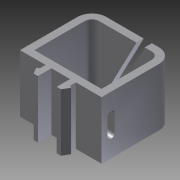
# Autodesk Inventor part: Cable V3
Saved by Autodesk Inventor 2012 (Build 160160000, 160)
## iProperties
Created: 2013-02-21
Part Number: Cable V3
Material: Default
Document SubType Name: Modeling
Designer: mce
Density: 1 g/cm^3
Author: mce
Autodesk Inventor part; units mm, degrees
ref_plane "YZ Plane" through (0, 0, 0) normal (1, 0, 0) x (0, 1, 0)
ref_plane "XZ Plane" through (0, 0, 0) normal (0, 1, 0) x (-1, 0, 0)
ref_plane "XY Plane" through (0, 0, 0) normal (0, 0, 1) x (1, 0, 0)
sketch "Sketch1" plane through (0, 0, 0) normal (0, 0, 1) x (1, 0, 0)
  line L0 (-0.3861, 13.3644) -> (-0.3861, 12.1644)
  line L1 (0.8139, 10.5644) -> (0.8139, 13.3644)
  line L2 (2.7639, 27.7657) -> (2.7639, 5.268) construction
  line L3 (-5.7361, 13.3644) -> (-5.7361, 25.3644)
  line L4 (-2.7361, 28.3644) -> (2.7639, 28.3644)
  line L5 (2.7639, 26.8644) -> (-2.7361, 26.8644)
  line L6 (-4.2361, 25.3644) -> (-4.2361, 14.8644)
  line L7 (-4.2361, 14.8644) -> (2.7639, 14.8644)
  line L8 (-0.3861, 12.1644) -> (-0.8539, 11.8943)
  line L9 (-5.7361, 13.3644) -> (-0.3861, 13.3644)
  arc A0 (-2.7361, 28.3644) -> (-5.7361, 25.3644) centre (-2.7361, 25.3644) ccw
  arc A1 (-2.7361, 26.8644) -> (-4.2361, 25.3644) centre (-2.7361, 25.3644) ccw
  line L10 (-0.8539, 11.8943) -> (-0.0861, 10.5644)
  line L11 (-0.0861, 10.5644) -> (0.8139, 10.5644)
  line L12 (5.6139, 10.5644) -> (4.7139, 10.5644)
  line L13 (11.2639, 13.3644) -> (11.2639, 25.3644)
  arc A2 (11.2639, 25.3644) -> (8.2639, 28.3644) centre (8.2639, 25.3644) ccw
  line L14 (8.2639, 28.3644) -> (2.7639, 28.3644)
  line L15 (2.7639, 26.8644) -> (8.2639, 26.8644)
  arc A3 (9.7639, 25.3644) -> (8.2639, 26.8644) centre (8.2639, 25.3644) ccw
  line L16 (9.7639, 25.3644) -> (9.7639, 14.8644)
  line L17 (9.7639, 14.8644) -> (2.7639, 14.8644)
  line L18 (11.2639, 13.3644) -> (5.9139, 13.3644)
  line L19 (5.9139, 13.3644) -> (5.9139, 12.1644)
  line L20 (5.9139, 13.3644) -> (6.9559, 13.3644)
  line L21 (4.7139, 10.5644) -> (4.7139, 13.3644)
  line L22 (6.3817, 11.8943) -> (5.6139, 10.5644)
  line L23 (5.9139, 12.1644) -> (6.3817, 11.8943)
  line L24 (0.8139, 13.3644) -> (4.7139, 13.3644)
  line L25 (5.9139, 13.3644) -> (6.9559, 13.3644)
  point P0 (0, 0)
  dimension "d1" = 1.2
  dimension "d2" = 1.95
  dimension "d3" = 120
  dimension "d5" = 8.5
  dimension "d6" = 1.5
  dimension "d8" = 1.5
  dimension "d9" = 12
  dimension "d10" = 3
  dimension "d11" = 1.5
  dimension "d12" = 0.9
  dimension "d13" = 120
  dimension "d15" = 1.2
  dimension "d16" = 2.8
  dimension "d17" = 1.5
  constraints: 52 end point, 14 symmetric about line, 8 point on circle, 4 centre point, 4 tangent, 3 horizontal, 3 point on line, 2 parallel, 2 vertical, 1 collinear, 1 perpendicular, 2 other
  measures "d1" distance between parallel lines of L0 L1
  measures "d2" distance between parallel lines of L2 L1
  measures "d3" angle of L0 L8
  measures "d5" distance between parallel lines of L2 L3
  measures "d6" distance between parallel lines of L3 L6
  measures "d8" distance between parallel lines of L4 L5
  measures "d9" distance between parallel lines of L5 L7
  measures "d10" radius of A0
  measures "d11" radius of A1
  measures "d12" distance of L11.start L1.start
  measures "d13" angle of L10 L11
  measures "d15" distance from line of L9 L8.start
  measures "d16" distance between parallel lines of L24 L11
  measures "d17" distance between parallel lines of L7 L9
extrude "Extrusion1" add sketch "Sketch1" along normal blind 12
sketch "Sketch2" plane through (-2.7361, 28.3644, 0) normal (0, 1, 0) x (1, 0, 0)
  line L0 (0, -12) -> (11, -12) projected
  line L1 (11, 0) -> (0, 0) projected
  line L2 (0, 0) -> (0, -12) projected
  line L3 (1.5, 0) -> (3.1945, 0)
  line L4 (3.1945, 0) -> (9.5, -12)
  line L5 (7.8055, -12) -> (1.5, 0)
  point P0 (2.7361, 0)
  dimension "d20" = 1.5
  dimension "d21" = 1.5
  dimension "d22" = 1.5
  constraints: 6 end point, 4 point on line, 1 parallel
  measures "d20" distance from line of L2 L3.start
  measures "d21" distance of L4.end L0.end
  measures "d22" distance between parallel lines of L5 L4
extrude "Extrusion2" cut sketch "Sketch2" against normal up to next contours L5 L1 L4 L0
sketch "Sketch3" plane through (11.2639, 13.3644, 0) normal (1, 0, 0) x (0, 0, -1)
  line L0 (-12, 12) -> (-12, 0) projected
  line L1 (0, 0) -> (-12, 0) projected
  arc A0 (-7.75, 2.75) -> (-7.75, 1.25) centre (-7.75, 2) ccw
  arc A1 (-4.25, 1.25) -> (-4.25, 2.75) centre (-4.25, 2) ccw
  line L2 (-7.75, 2.75) -> (-4.25, 2.75)
  line L3 (-4.25, 1.25) -> (-7.75, 1.25)
  point P0 (0, -13.3644)
  dimension "d30" = 1.5
  dimension "d31" = 3.5
  dimension "d32" = 4.25
  dimension "d33" = 2
  constraints: 4 end point, 4 point on circle, 4 vertical alignment, 2 centre point, 1 equal radius, 1 horizontal alignment
  measures "d30" diameter of A0
  measures "d31" distance of A1.centre A0.centre
  measures "d32" distance from line of L0 A0.centre
  measures "d33" distance from line of L1 A0.centre
extrude "Extrusion3" cut sketch "Sketch3" against normal through all
body "Solid1"
